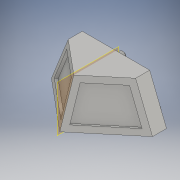
# Autodesk Inventor part: Caufield_Cow_Catcher
Saved by Autodesk Inventor 2016 (Build 200138000, 138)
## iProperties
Created: 2018-01-16
Part Number: Caufield_Cow_Catcher
Material: Generic
Document SubType Name: Modeling
Designer: caufield58738
Density: 1 g/cm^3
Appearance: Default
Mass: 4.36656 g
Surface Area: 45.1722 cm^2
Volume: 4.36656 cm^3
Author: caufield58738
Autodesk Inventor part; units mm, degrees
ref_plane "YZ Plane" through (0, 0, 0) normal (1, 0, 0) x (0, 1, 0)
ref_plane "XY Plane" through (0, 0, 0) normal (0, 0, 1) x (1, 0, 0)
sketch "Sketch1" plane through (0, 0, 0) normal (0, 1, 0) x (-1, 0, 0)
  line L0 (0, 0) -> (0, -22.86)
  line L1 (0, -22.86) -> (6.35, -22.86)
  line L2 (6.35, -22.86) -> (25.4, -22.86) construction
  line L3 (25.4, -22.86) -> (25.4, 0) construction
  line L4 (6.35, -22.86) -> (25.4, 0)
  line L5 (25.4, 0) -> (0, 0) construction
  line L6 (0, 0) -> (0, 22.86)
  line L7 (0, 22.86) -> (6.35, 22.86)
  line L8 (6.35, 22.86) -> (25.4, 0)
  dimension "d0" = 22.86
  dimension "d1" = 6.35
  dimension "d2" = 19.05
  dimension "d3" = 25.4
  constraints: 18 end point, 2 perpendicular, 2 symmetric about line, 1 point on line, 1 vertical
  measures "d0" distance of L0.start L0.end
  measures "d1" distance of L0.end L1.end
  measures "d2" distance of L1.end L2.end
  measures "d3" distance of L0.start L3.end
ref_plane "Work Plane1" through (0, 19.05, 0) normal (0, 1, 0) x (-1, 0, 0)
sketch "Sketch2" plane through (0, 19.05, 0) normal (0, 1, 0) x (-1, 0, 0)
  line L0 (0, 0) -> (0, -15.24)
  line L1 (0, -15.24) -> (6.35, -15.24)
  line L2 (6.35, -15.24) -> (19.05, -15.24) construction
  line L3 (19.05, -15.24) -> (19.05, 0) construction
  line L4 (19.05, 0) -> (0, 0) construction
  line L5 (19.05, 0) -> (6.35, -15.24)
  line L6 (0, 0) -> (0, 15.24)
  line L7 (0, 15.24) -> (6.35, 15.24)
  line L8 (19.05, 0) -> (6.35, 15.24)
  dimension "d5" = 15.24
  dimension "d6" = 6.35
  dimension "d7" = 12.7
  constraints: 18 end point, 3 perpendicular, 2 symmetric about line, 1 point on line, 1 vertical
  measures "d5" distance of L0.start L0.end
  measures "d6" distance of L0.end L1.end
  measures "d7" distance of L1.end L2.end
loft "Loft1" add profiles "Sketch1", "Sketch2"
shell "Shell1" thickness 2.54 removed faces 1 at (-10.5833, 0, 7.62)
sketch "Sketch4" plane through (-25.4, 0, 0) normal (-0.7442084, 0.2480695, 0.6201737) x (0.6401844, 0, 0.7682213)
  line L0 (6.1338, 17.1247) -> (3.1188, 2.54)
  line L1 (3.1188, 2.54) -> (26.3508, 2.54)
  line L2 (26.3508, 2.54) -> (22.0092, 17.1247)
  line L3 (22.0092, 17.1247) -> (6.1338, 17.1247)
  line L4 (0, 0) -> (29.7571, 0) projected
  line L5 (29.7571, 0) -> (23.9032, 19.6647) projected
  line L6 (4.0652, 19.6647) -> (23.9032, 19.6647) projected
  line L7 (0, 0) -> (4.0652, 19.6647) projected
  line L8 (29.7571, 0) -> (23.9032, 19.6647) projected
  dimension "d13" = 2.54
  dimension "d14" = 2.54
  dimension "d15" = 2.54
  dimension "d16" = 2.54
  constraints: 8 end point, 4 parallel, 1 horizontal
  measures "d13" distance between parallel lines of L7 L0
  measures "d14" distance between parallel lines of L3 L6
  measures "d15" distance between parallel lines of L5 L2
  measures "d16" distance between parallel lines of L4 L1
extrude "Extrusion1" cut sketch "Sketch4" against normal blind 1.27 contours L3 L2 L1 L0
ref_plane "Work Plane2" through (-6.35, 57.15, 0) normal (0, 0, 1) x (1, 0, 0)
mirror "Mirror1" about plane through (-6.35, 57.15, 0) normal (0, 0, 1) of "Extrusion1"
sketch "Sketch5" plane through (0, 0, 22.86) normal (1, 0, 0) x (0, 0, -1)
  circle A0 centre (6.985, 3.175) radius 1.5875
  circle A1 centre (22.86, 15.875) radius 1.5875
  line L0 (0, 0) -> (45.72, 0) projected
  line L1 (22.86, 0) -> (22.86, 19.05) construction
  line L2 (22.86, 19.05) -> (22.86, 0) construction
  circle A2 centre (38.735, 3.175) radius 1.5875
  dimension "d19" = 3.175
  dimension "d20" = 3.175
  dimension "d21" = 3.175
  dimension "d22" = 6.985
  dimension "d23" = 15.875
  dimension "d24" = 45.72
  dimension "d25" = 22.86
  constraints: 3 centre point, 2 end point, 1 symmetric about line, 1 vertical, 1 other
  measures "d19" diameter of A0
  measures "d20" diameter of A1
  measures "d21" distance from line of L0 A0.centre
  measures "d22" horizontal distance of L0.start A0.centre
  measures "d23" distance from line of L0 A1.centre
  measures "d24" distance of L0.end L0.start
  measures "d25" horizontal distance of L0.end A1.centre
extrude "Extrusion3" add sketch "Sketch5" along normal blind 3.175
chamfer "Chamfer2" distance 0.254 angle 45 3 edges at (3.175, 15.875, 1.5875) (3.175, 3.175, 17.4625) (3.175, 3.175, -14.2875)
body "Solid1"
